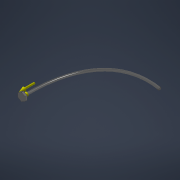
# Autodesk Inventor part: large_hoop
Saved by Autodesk Inventor 2021 (Build 250183000, 183)
## iProperties
Created: 2021-05-05
Part Number: large_hoop
Material: Steel C350L0
Document SubType Name: Modeling
Density: 7.85 g/cm^3
Appearance: Steel C350L0
Mass: 7260.78 g
Surface Area: 3505.54 cm^2
Volume: 924.94 cm^3
Autodesk Inventor part; units mm, degrees
ref_plane "YZ Plane" through (0, 0, 0) normal (1, 0, 0) x (0, 1, 0)
ref_plane "XZ Plane" through (0, 0, 0) normal (0, 1, 0) x (-1, 0, 0)
sketch "Sketch1" plane through (0, 0, 0) normal (1, 0, 0) x (0, 1, 0)
  circle A0 centre (0, 0) radius 1650
  dimension "d0" = 3300
  constraints: 1 centre point, 1 coincident
  measures "d0" diameter of A0
sketch "Sketch2" plane through (0, 0, 0) normal (0, 0, 1) x (1, 0, 0)
  circle A0 centre (0, 1650) radius 12.7
  point P0 (0, 0)
  dimension "d1" = 1650
  dimension "d2" = 0
  dimension "d3" = 25.4
  constraints: 1 centre point
  measures "d1" distance of A0.centre point (0, 0)
  measures "d2" horizontal distance of A0.centre point (0, 0)
  measures "d3" diameter of A0
sweep "Sweep1" add profiles "Sketch2" path "Sketch1"
sketch "Sketch3" plane through (0, 0, 0) normal (0, 0, 1) x (1, 0, 0)
  circle A0 centre (0, 1650) radius 11.7
  point P0 (0, 0)
  dimension "d6" = 23.4
  dimension "d7" = 0
  dimension "d8" = 1650
  constraints: 1 centre point
  measures "d6" diameter of A0
  measures "d7" horizontal distance of A0.centre point (0, 0)
  measures "d8" distance of point (0, 0) A0.centre
sweep "Sweep2" cut profiles "Sketch3" path "Sketch1"
sketch "Sketch4" plane through (0, 0, 0) normal (1, 0, 0) x (0, 1, 0)
  line L0 (1050, 1701) -> (1050, -1701)
  line L1 (1050, 51) -> (2751, 51)
  line L2 (2751, 51) -> (2751, 1701)
  line L3 (1050, 1701) -> (1180.0646, 1701)
  line L4 (1180.0646, 1701) -> (2751, 1701)
  line L5 (1050, 1701) -> (-1701, 1701)
  line L6 (-1701, 1701) -> (-1701, -1701)
  line L7 (-1701, -1701) -> (1050, -1701)
  point P0 (0, 0)
  dimension "d12" = 3402
  dimension "d13" = 1701
  dimension "d14" = 1050
  dimension "d15" = 1701
  dimension "d16" = 1701
  dimension "d17" = 51
  constraints: 17 end point, 2 horizontal, 2 perpendicular, 2 point on line, 2 vertical
  measures "d12" distance of L0.start L0.end
  measures "d13" vertical distance of point (0, 0) L0.start
  measures "d14" distance from line of point (0, 0) L0
  measures "d15" distance from line of point (0, 0) L6
  measures "d16" distance of L1.start L1.end
  measures "d17" distance from line of point (0, 0) L1
extrude "Extrusion1" cut sketch "Sketch4" along normal mid plane 51
sketch "Sketch5" plane through (0, 1050, -1272.7491) normal (0, -1, 0) x (1, 0, 0)
  line L0 (3.5, -4.2386) -> (-3.5, -4.2386)
  line L1 (-3.5, -4.2386) -> (-3.5, 41.1701)
  line L2 (-3.5, 41.1701) -> (3.5, 41.1701)
  line L3 (3.5, 41.1701) -> (3.5, -4.2386)
  line L4 (0, 1591.7945) -> (0, -284.51) projected
  point P0 (0, 1272.7491)
  dimension "d20" = 7
  dimension "d21" = 3.5
  constraints: 8 end point, 2 parallel, 1 horizontal, 1 perpendicular
  measures "d20" distance between parallel lines of L1 L3
  measures "d21" distance between parallel lines of L4 L1
extrude "Extrusion2" cut sketch "Sketch5" against normal blind 5
fillet "Fillet2" [suppressed]
ref_plane "Work Plane1" through (0, 0, -1250) normal (0, 0, 1) x (1, 0, 0)
sketch "Sketch6" plane through (0, 1649.2116, 51) normal (0, 0, 1) x (1, 0, 0)
  line L0 (0, 378.3261) -> (0, -1987.1345) projected
  line L1 (0, 40.4032) -> (-34.641, 20.4032)
  line L2 (-34.641, 20.4032) -> (-34.641, -19.5968)
  line L3 (-34.641, -19.5968) -> (0, -39.5968)
  line L4 (0, -39.5968) -> (34.641, -19.5968)
  line L5 (34.641, -19.5968) -> (34.641, 20.4032)
  line L6 (34.641, 20.4032) -> (0, 40.4032)
  point P0 (0, -1649.2116)
  dimension "d32" = 120
  dimension "d33" = 120
  dimension "d34" = 40
  dimension "d35" = 120
  dimension "d36" = 120
  dimension "d37" = 120
  constraints: 12 end point, 3 equal length, 1 point on line, 1 vertical
  measures "d32" angle of L1 L2
  measures "d33" angle of L2 L3
  measures "d34" distance of L1.end L2.end
  measures "d35" angle of L5 L4
  measures "d36" angle of L6 L5
  measures "d37" angle of L4 L3
extrude "Extrusion4" add sketch "Sketch6" along normal blind 20
sketch "Sketch7" plane through (0, 0, 0) normal (1, 0, 0) x (0, 1, 0)
  circle A0 centre (0, 0) radius 1650
  line L0 (1038.8958, -1282.1092) -> (1115.6409, -1217.9985)
  line L1 (1050, -1256.9256) -> (1050, -1258.2856) projected
  line L2 (1050, -1256.9256) -> (1094.326, -1309.987)
  line L3 (1050, -1256.9256) -> (1029.6814, -1273.8992)
  line L4 (1029.6814, -1273.8992) -> (1029.6814, -1346.8295)
  line L5 (1029.6814, -1346.8295) -> (1094.326, -1309.987)
  point P0 (1057.8268, -1266.2948)
  dimension "d40" = 3300
  dimension "d41" = 100
  constraints: 10 end point, 2 perpendicular, 2 point on line, 1 coincident, 1 vertical, 4 other
  measures "d41" distance of L0.start L0.end
extrude "Extrusion5" cut sketch "Sketch7" against normal mid plane 100 contours L4 L3 L2 A0 | A0 L2 L5 L4 picked at (1042.7276, -1268.2839)
sketch "Sketch10" plane through (0, 1057.8268, -1266.2948) normal (0, -0.7674514, -0.6411071) x (1, 0, 0)
  line L0 (3.5, 11.1642) -> (3.5, 12.2082) projected
  line L1 (-3.5, 12.2082) -> (-3.5, 11.1642) projected
  line L2 (3.5, 11.1642) -> (-3.5, 11.1642)
  line L3 (-3.5, 11.1642) -> (-3.5, 12.2082)
  line L4 (-3.5, 12.2082) -> (3.5, 12.2082)
  line L5 (3.5, 12.2082) -> (3.5, 11.1642)
  point P0 (0, 1650)
  point P1 (3.5, 14.586)
  point P2 (-3.5, 14.586)
  constraints: 8 end point, 2 parallel, 1 horizontal, 1 perpendicular
extrude "Extrusion6" cut sketch "Sketch10" against normal blind 10
fillet "Fillet3" [suppressed]
sketch "Sketch11" plane through (0, 1057.8268, -1266.2948) normal (0, -0.7674514, -0.6411071) x (1, 0, 0)
  circle A0 centre (0, 0) radius 14.7
  arc A1 (-3.5, 11.1642) -> (3.5, 11.1642) centre (0, 0) ccw projected
  line L0 (-3.5, 11.1849) -> (-3.5, 11.1642) projected
  arc A2 (3.5, 11.1642) -> (-3.5, 11.1642) centre (0, 0) ccw
  point P0 (0, 1650)
  point P1 (-3.5, 11.174)
  dimension "d60" = 3
  constraints: 2 centre point, 2 point on circle, 1 coincident, 1 concentric
  measures "d60" radial gap between concentric circles of A0 A1
extrude "Extrusion9" add sketch "Sketch11" along normal blind 10
sketch "Sketch13" plane through (0, 1050.1522, -1272.7059) normal (0, -0.7674514, -0.6411071) x (1, 0, 0)
  line L0 (-3.5, 12.2082) -> (-3.5, 11.1642) projected
  line L1 (-3.5, 9.5915) -> (3.5, 9.5915)
  line L2 (3.5, 9.5915) -> (3.5, 21.2168)
  line L3 (3.5, 21.2168) -> (-3.5, 21.2168)
  line L4 (-3.5, 21.2168) -> (-3.5, 9.5915)
  point P0 (0, 1650)
  point P1 (-3.5, 19.0616)
  point P2 (-3.5, 19.0616)
  point P3 (-3.5, 12.2082)
  point P4 (-3.5, 11.1642)
  dimension "d55" = 7
  constraints: 8 end point, 2 parallel, 1 horizontal, 1 perpendicular, 1 point on line
  measures "d55" distance of L2.end L3.end
extrude "Extrusion10" cut sketch "Sketch13" against normal blind 10
fillet "Fillet6" radius 1 2 edges at (10.1425, 1052.9266, -1260.4289) (-7.6432, 1064.3292, -1274.0787)
ref_plane "Work Plane2" through (0, 1180.619, -1163.7177) normal (0, -0.7674514, -0.6411071) x (1, 0, 0)
split "Split1" [suppressed]
equation "\"d0\" = hoop_radius_large"
equation "\"d1\" = 0.5 * d0"
equation "\"d3\" = hoop_width_small"
equation "\"d6\" = hoop_width_small - hoop_thickness_small"
equation "\"d8\" = 0.5 * d0"
equation "\"d12\" = 2 * hoop_width_large + d0"
equation "\"d13\" = 0.5 * d12"
equation "\"d14\" = 0.5 * hoop_radius_large - hoop_height_small"
equation "\"d15\" = 0.5 * d12"
equation "\"d16\" = d13"
equation "\"d17\" = hoop_width_large"
equation "\"d18\" = hoop_width_large"
equation "\"d21\" = 0.5 * d20"
equation "\"d22\" = hoop_cable_diam"
equation "\"d40\" = hoop_radius_large"
equation "\"hoop_radius_large\" = 3300"
equation "\"hoop_width_large\" = 51"
equation "\"d11\" = 2 * hoop_width_large + 0.5 * d0"
equation "\"hoop_thickness_small\" = 2"
equation "\"hoop_width_small\" = 25.4"
equation "\"hoop_cable_diam\" = 5"
equation "\"hoop_angle_z\" = 45deg"
equation "\"hoop_bearing_length\" = 5deg"
equation "\"hoop_cable_pulley_diam\" = 22"
equation "\"hoop_thickness_large\" = 4"
equation "\"hoop_thickness_medium\" = 3.2"
equation "\"hoop_width_medium\" = 33.7"
equation "\"hoop_bushing12_od\" = -2 * hoop_thickness_large + hoop_width_large + hoop_bushing12_radialInterference"
equation "\"hoop_bushing12_radialInterference\" = 0"
equation "\"hoop_bushing12_thickness\" = -hoop_width_medium + hoop_bushing12_od - 2 * hoop_bushing12_radialInterference"
equation "\"hoop_bushing23_od\" = -2 * hoop_thickness_medium + hoop_width_medium + hoop_bushing23_radialInterference"
equation "\"hoop_bushing23_radialInterference\" = 0"
equation "\"hoop_bushing23_thickness\" = -hoop_width_small + hoop_bushing23_od - 2 * hoop_bushing23_radialInterference"
equation "\"hoop_tabs_hole\" = 12"
equation "\"hoop_tabs_thickness\" = 6"
equation "\"rack_tooth_addendum\" = 5"
equation "\"rack_tooth_dedendum\" = 5"
equation "\"rack_tooth_thickness\" = 5"
equation "\"secure_arm_angle\" = 35deg"
equation "\"secure_arm_radii\" = 9"
equation "\"sm_varx_member_tolerance\" = 0.5"
equation "\"sm_varx_pinPlate_holeDiameter\" = 5"
equation "\"sm_varx_pinPlate_thickness\" = 5"
equation "\"sm_varx_squareBarThickness\" = 2.5"
equation "\"support_baseClamp_platformLengthBuffer\" = 35"
equation "\"support_baseClamp_platformThickness\" = 15"
equation "\"support_baseClamp_platformWidthBuffer\" = 0"
equation "\"support_baseClamp_sleeveHoleDiameter\" = 12"
equation "\"support_baseClamp_sleeveSweepTerminationAngle\" = 55deg"
equation "\"support_baseClamp_thickness\" = 8"
equation "\"support_frame_endHoleBuffer\" = 25"
equation "\"support_frame_squareBarFillet\" = 2"
equation "\"support_frame_squareBarThickness\" = 5"
equation "\"wheelchair_deployed_height\" = 914"
equation "\"wheelchair_deployed_length\" = 1067"
equation "\"wheelchair_deployed_width\" = 635"
equation "\"hoop_height_small\" = 600"
body "Solid1"
body "Solid2"
body "Solid3"
